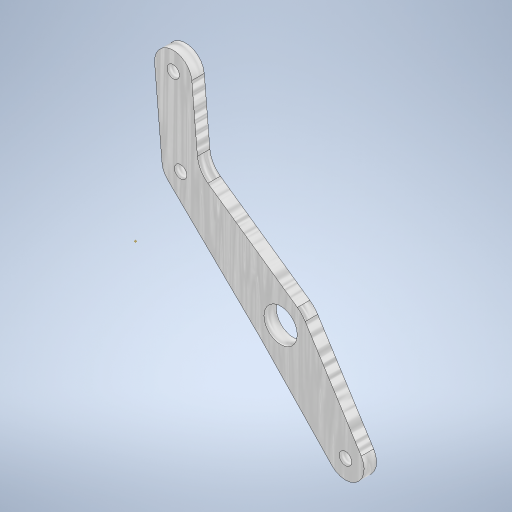
# Autodesk Inventor part: アーノン
Saved by Autodesk Inventor 2023 (Build 270158000, 158)
## iProperties
Created: 2022-01-29
Part Number: アーノン
Material: Aluminum 7075
Document SubType Name: Modeling
Designer: acps
Density: 2.81 g/cm^3
Appearance: Satin - Brushed Heavy
Author: acps
Autodesk Inventor part; units mm, degrees
ref_plane "YZ Plane" through (0, 0, 0) normal (1, 0, 0) x (0, 1, 0)
ref_plane "XZ Plane" through (0, 0, 0) normal (0, 1, 0) x (-1, 0, 0)
ref_plane "XY Plane" through (0, 0, 0) normal (0, 0, 1) x (1, 0, 0)
sketch "Sketch2" plane through (0, 0, 0) normal (0, 0, 1) x (1, 0, 0)
  circle A0 centre (9.1116, 40) radius 1.5
  circle A1 centre (9.1116, 40) radius 4.5
  circle A2 centre (35, 0) radius 4.025
  circle A3 centre (35, 0) radius 7.025
  circle A4 centre (10.8954, 20) radius 1.5
  circle A5 centre (10.8954, 20) radius 4.5
  circle A6 centre (50.6355, -20) radius 1.5
  circle A7 centre (50.6355, -20) radius 4.5
  arc A8 (28.8107, -1.9856) -> (20.579, 14.4531) centre (-28.3213, -20.3142) ccw construction
  arc A9 (18.0263, 45.1752) -> (16.1159, 20.406) centre (30.0598, 31.7888) ccw construction
  arc A10 (18.0263, 45.1752) -> (18.7829, 48.816) centre (15.9272, 47.5104) ccw construction
  arc A11 (20.496, 56.1256) -> (18.7829, 48.816) centre (24.3578, 51.365) ccw construction
  arc A12 (49.7418, -14.1257) -> (33.14, -6.2282) centre (15.9708, -63.7192) ccw construction
  arc A13 (52.5589, -35.9867) -> (51.8531, -15.4268) centre (46.0292, -25.9188) ccw construction
  arc A14 (49.7418, -14.1257) -> (51.8531, -15.4268) centre (65.07, 8.3841) ccw construction
  line L0 (20.9971, 13.8809) -> (15.6661, 20.9804) construction
  line L1 (39.0353, 5.7504) -> (13.4803, 23.6835)
  line L2 (30.093, -5.0271) -> (7.7521, 16.7798)
  line L3 (6.4132, 19.6002) -> (4.6294, 39.6002)
  line L4 (13.5938, 40.3998) -> (15.3776, 20.3998)
  line L5 (40.9374, 3.7548) -> (54.4388, -17.5948)
  line L6 (30.2382, -5.185) -> (47.3835, -23.1104)
  arc A15 (14.9442, 25.2593) -> (17.4739, 20.881) centre (20.9205, 25.7924) ccw
  arc A16 (30.2382, -5.185) -> (30.093, -5.0271) centre (28.696, -6.4584) ccw
  point P0 (0, 0)
  point P1 (15.1918, 22.4824)
  dimension "d25" = 3
  dimension "d26" = 9
  dimension "d27" = 8.05
  dimension "d28" = 14.05
  dimension "d29" = 3
  dimension "d30" = 9
  dimension "d31" = 3
  dimension "d32" = 9
  dimension "d33" = 40
  dimension "d34" = 20
  dimension "d35" = 20
  dimension "d36" = 6
  dimension "d37" = 2
  constraints: 28 point on circle, 19 tangent, 17 centre point, 14 end point, 5 coincident, 2 point on line, 10 other
  measures "d25" diameter of A0
  measures "d26" diameter of A1
  measures "d27" diameter of A2
  measures "d28" diameter of A3
  measures "d29" diameter of A4
  measures "d30" diameter of A5
  measures "d31" diameter of A6
  measures "d32" diameter of A7
  measures "d33" vertical distance of point (0, 0) A0.centre
  measures "d34" vertical distance of point (0, 0) A4.centre
  measures "d35" vertical distance of A6.centre point (0, 0)
  measures "d36" radius of A15
  measures "d37" radius of A16
extrude "Extrusion2" add sketch "Sketch2" against normal blind 3
body "Solid2"
